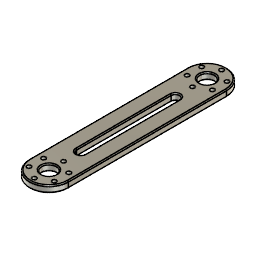
Arm Link v5 (Autodesk Fusion 360 design; units mm, degrees)
Autodesk Fusion 360 part; units mm, degrees
sketch "Sketch1" plane through (0, 0, 0) normal (0, 0, 1) x (1, 0, 0)
  line L0 (0, 0) -> (0, 100)
  line L1 (0, 0) -> (0, 80)
  circle A0 centre (0, 80) radius 15
  circle A1 centre (0, 95) radius 2.15
  circle A2 centre (-12.9904, 87.5) radius 2.15
  circle A3 centre (-12.9904, 72.5) radius 2.15
  circle A4 centre (0, 65) radius 2.15
  circle A5 centre (12.9904, 72.5) radius 2.15
  circle A6 centre (12.9904, 87.5) radius 2.15
  circle A7 centre (0, 80) radius 20
  line L2 (0, 80) -> (-20, 80)
  line L3 (0, 80) -> (20, 80)
  line L4 (-20, 80) -> (20, 80)
  line L5 (20, 80) -> (20, -1.3686)
  line L6 (20, -1.3686) -> (-20, -1.3686)
  line L7 (-20, -1.3686) -> (-20, 80)
  circle A8 centre (0, 47.2628) radius 4.3103
  line L8 (0, 47.2628) -> (-4.3103, 47.2628)
  line L9 (0, 47.2628) -> (4.3103, 47.2628)
  line L10 (-4.3103, 47.2628) -> (4.3103, 47.2628)
  line L11 (4.3103, 47.2628) -> (4.3103, -33.1681)
  line L12 (4.3103, -33.1681) -> (-4.3103, -33.1681)
  line L13 (-4.3103, -33.1681) -> (-4.3103, 47.2628)
  line L14 (-20, -1.3686) -> (-20, -82.7372)
  circle A9 centre (0, -97.7372) radius 2.15
  line L15 (0, -2.7372) -> (0, -82.7372)
  line L16 (0, -82.7372) -> (-20, -82.7372)
  line L17 (20, -82.7372) -> (20, -1.3686)
  circle A10 centre (-12.9904, -90.2372) radius 2.15
  line L18 (0, -2.7372) -> (0, -102.7372)
  line L19 (-4.3103, -50) -> (4.3103, -50)
  line L20 (4.3103, -50) -> (4.3103, 30.4309)
  circle A11 centre (12.9904, -75.2372) radius 2.15
  line L21 (0, -50) -> (-4.3103, -50)
  line L22 (-20, -82.7372) -> (20, -82.7372)
  circle A12 centre (0, -82.7372) radius 20
  line L23 (-4.3103, 30.4309) -> (-4.3103, -50)
  line L24 (20, -1.3686) -> (-20, -1.3686)
  line L25 (0, -50) -> (4.3103, -50)
  circle A13 centre (0, -50) radius 4.3103
  line L26 (4.3103, 30.4309) -> (-4.3103, 30.4309)
  circle A14 centre (0, -67.7372) radius 2.15
  circle A15 centre (-12.9904, -75.2372) radius 2.15
  circle A16 centre (0, -82.7372) radius 15
  line L27 (0, -82.7372) -> (20, -82.7372)
  circle A17 centre (12.9904, -90.2372) radius 2.15
  circle A18 centre (0, 80) radius 7.5
  circle A19 centre (0, -82.7372) radius 7.5
  point P0 (0, -2.7372)
  dimension "d6" = 100
  dimension "d7" = 80
  dimension "d8" = 30
  dimension "d9" = 4.3
  dimension "d11" = 360
  dimension "d18" = 15
  dimension "d21" = 15
  constraint coincident L0.start L1.start
  constraint vertical L0
  constraint parallel L0 L1
  constraint coincident L1.end A0.centre
  constraint coincident A0 A1.centre
  constraint coincident L0 A1.centre
  constraint concentric A0 A7
  constraint coincident L0.end A7
  constraint coincident A7 L2.end
  constraint perpendicular L1 L2
  constraint coincident A7 L3.end
  constraint parallel L2 L3
  constraint perpendicular L4 L5
  constraint parallel L4 L6
  constraint parallel L5 L7
  constraint coincident L1 A8.centre
  constraint coincident A8.centre L8.start
  constraint coincident A8 L8.end
  constraint perpendicular L0 L8
  constraint coincident A8 L9.end
  constraint perpendicular L0 L9
  constraint perpendicular L10 L11
  constraint parallel L10 L12
  constraint parallel L11 L13
  constraint symmetric L0.start L6 L15.start
  constraint symmetric L0.start L6 P0
  constraint symmetric L0.end L6 L18.end
  constraint symmetric L1.end L6 L15.end
  constraint symmetric A0 L6 A16
  constraint symmetric A1 L6 A9
  constraint symmetric A2 L6 A10
  constraint symmetric A3 L6 A15
  constraint symmetric A4 L6 A14
  constraint symmetric A5 L6 A11
  constraint symmetric A6 L6 A17
  constraint symmetric A7 L6 A12
  constraint symmetric L2.end L6 L14.end
  constraint symmetric L3.end L6 L17.start
  constraint symmetric L5.end L6 L17.end
  constraint symmetric L7.start L6 L14.start
  constraint symmetric L6 A8 A13
  constraint symmetric L6 A8.centre L21.start
  constraint symmetric L6 L8.end L19.start
  constraint symmetric L6 L9.end L19.end
  constraint symmetric L6 L11.end L20.end
  constraint symmetric L6 L12.end L23.start
  constraint coincident L21.start L25.start
  constraint concentric A7 A18
  constraint coincident L15.end L16.start
  measures "d6" distance of L0.start L0.end
  measures "d7" distance of L0.start L1.end
  measures "d8" diameter of A0
  measures "d9" diameter of A1
  measures "d18" diameter of A19
  measures "d21" diameter of A18
extrude "Extrude1" add sketch "Sketch1" along normal blind 7 contours L0 L1 A7 L5 L6 A8 L11 L20 L24 | L0 L1 A7 L6 L7 A8 L13 L23 L24 | L6 L11 L15 L17 L18 L20 A12 L24 A13 | L6 L13 L14 L15 L18 A12 L23 L24 A13 | L0 L1 A0 A3 A4 A7 L2 L4 | L0 L1 A0 A4 A5 A7 L3 L4 | L0 A0 A1 A6 A7 L3 L4 | A9 L18 L22 A12 A16 L27 A17 | L15 L18 A11 L22 A12 A14 A16 L27 | L0 A0 A1 A2 A7 L2 L4 | L15 L16 L18 L22 A12 A14 A15 A16 | A9 L16 A10 L18 L22 A12 A16 | L0 A0 A1 A6 L3 L4 A18 | L0 L1 A0 A4 A5 L3 L4 A18 | A9 L18 L22 A16 L27 A17 A19 | L15 L18 A11 L22 A14 A16 L27 A19 | L0 L1 A0 A3 A4 L2 L4 A18 | L0 A0 A1 A2 L2 L4 A18 | L15 L16 L18 L22 A14 A15 A16 A19 | A9 L16 A10 L18 L22 A16 A19
fillet "Fillet1" radius 1 8 edges at (20, -1.3686, 7) (0, 100, 7) (-20, -1.3686, 7) (0, -102.7372, 7) (0, 100, 0) (20, -1.3686, 0) (0, -102.7372, 0) (-20, -1.3686, 0)
fillet "Fillet2" radius 1 8 edges at (-4.3103, -1.3686, 7) (0, 51.5732, 7) (4.3103, -1.3686, 7) (0, -54.3103, 7) (4.3103, -1.3686, 0) (0, -54.3103, 0) (-4.3103, -1.3686, 0) (0, 51.5732, 0)
fillet "Fillet3" radius 1 4 edges at (-6.9925, 82.7121, 7) (-6.9925, 82.7121, 0) (-6.9925, -80.0251, 7) (-6.9925, -80.0251, 0)
